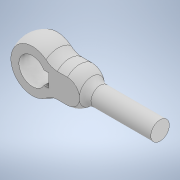
# Autodesk Inventor part: 1_3
Saved by Autodesk Inventor 2020.1 (Build 241239000, 239)
## iProperties
Created: 2022-02-23
Part Number: 1_3
Material: Типовые
Document SubType Name: Modeling
Designer: User
Density: 1 g/cm^3
Appearance: По умолчанию
Author: User
Autodesk Inventor part; units mm, degrees
ref_plane "YZ Plane" through (0, 0, 0) normal (1, 0, 0) x (0, 1, 0)
ref_plane "XZ Plane" through (0, 0, 0) normal (0, 1, 0) x (-1, 0, 0)
ref_plane "XY Plane" through (0, 0, 0) normal (0, 0, 1) x (1, 0, 0)
sketch "Эскиз1" plane through (0, 0, 0) normal (0, 0, 1) x (1, 0, 0)
  circle A0 centre (0, 0) radius 60
  circle A1 centre (0, 0) radius 32.5
  line L0 (28.2887, 16) -> (28.2887, -16)
  line L1 (28.2887, 16) -> (39.5, 16)
  line L2 (39.5, 16) -> (39.5, -16)
  line L3 (39.5, -16) -> (28.2887, -16)
  line L4 (-60, 0) -> (279.451, 0)
  line L5 (42.8486, 42) -> (42.8486, -42)
  line L6 (42.8486, 42) -> (85, 42)
  line L7 (85, 42) -> (85, -42)
  line L8 (85, -42) -> (42.8486, -42)
  line L9 (42.8486, -42) -> (42.8486, 42)
  circle A2 centre (60.2993, 92) radius 50
  line L10 (0, 0) -> (60.2993, 92)
  circle A3 centre (85, 0) radius 42
  line L11 (85, 22.5) -> (278.9533, 22.5)
  line L12 (278.9533, 22.5) -> (278.9533, -22.5)
  line L13 (278.9533, -22.5) -> (85, -22.5)
  line L14 (85, -22.5) -> (85, 22.5)
  circle A4 centre (134.2722, 52.5) radius 30
  line L15 (85, 0) -> (134.2722, 52.5)
  point P0 (-32.5, 0)
  point P1 (278.9533, 0)
  point P2 (278.9533, 0)
  point P3 (134.2722, 22.5)
  point P4 (113.7421, 30.625)
  point P5 (60.2993, 42)
  point P6 (32.8905, 50.1818)
  dimension "d17" = 84
  dimension "d0" = 120
  dimension "d1" = 65
  dimension "d2" = 32
  dimension "d3" = 72
  dimension "d4" = 84
  dimension "d7" = 100
  dimension "d8" = 92
  dimension "d10" = 110
  dimension "d11" = 85
  dimension "d12" = 0
  dimension "d13" = 45
  dimension "d14" = 60
  dimension "d15" = 52.5
  dimension "d16" = 72
  dimension "d18" = 0
  constraints: 32 end point, 6 point on circle, 5 horizontal, 5 parallel, 4 centre point, 4 perpendicular, 2 coincident, 2 midpoint, 2 point on line, 1 vertical, 3 other
  measures "d0" diameter of A0
  measures "d1" diameter of A1
  measures "d2" distance of L0.start L0.end
  measures "d3" horizontal distance of point (-32.5, 0) L1.end
  measures "d4" distance of L5.start L5.end
  measures "d7" diameter of A2
  measures "d8" distance from line of L4 L10.end
  measures "d10" distance of L10.start L10.end
  measures "d11" horizontal distance of L7.end point (0, 0)
  measures "d12" distance from line of L4 point (278.953, 0)
  measures "d13" distance of L11.end L12.end
  measures "d14" diameter of A4
  measures "d15" distance from line of L4 L15.end
  measures "d16" distance of L15.start L15.end
  measures "d18" distance of point (85, 0) L15.start
revolve "Вращение1" add sketch "Эскиз1" angle 360 about axis through (-60, 0, 0) along (1, 0, 0) picked at (45.8038, 26.0598) picked at (54.3043, 5.6582) picked at (76.4143, 10.6672) picked at (29.0608, 8.9784) contours A0 L10 A1 L4 | A2 L6 A0 | A0 L5 L4 L2 L1 A1 L10 | A1 L10 L4 | L5 A0 A3 L4 | L6 A3 A0 | A1 L0 L4 L10 | L4 A3 A0 | A0 A3 L7 L4 | L4 A1 L1 L2 | A3 L15 L11 L7 | A1 L4 L0 | L15 L11 A3 L4 | L7 L11 L15 | A3 L11 L12 L4 | A4 L11 A3 | A3 L11 L15
sketch "Эскиз2" plane through (0, 0, 0) normal (0, 1, 0) x (-1, 0, 0)
  line L0 (105.3756, -30) -> (-295.1428, -30)
  line L1 (-295.1428, -30) -> (-295.1428, 30)
  line L2 (-295.1428, 30) -> (105.3756, 30)
  line L3 (105.3756, 30) -> (105.3756, -30)
  point P0 (0, 0)
  point P1 (105.3756, 0)
  point P2 (0, 0)
  dimension "d20" = 0
  dimension "d21" = 60
  constraints: 8 end point, 2 parallel, 1 coincident, 1 horizontal, 1 midpoint, 1 perpendicular
  measures "d20" vertical distance of point (105.376, 0) point (0, 0)
  measures "d21" distance of L2.end L0.start
extrude "Выдавливание1" cut sketch "Эскиз2" along normal mid plane 200 keep common part
sketch "Эскиз3" plane through (60.2993, -29.3939, 30) normal (0, 0, 1) x (1, 0, 0)
  circle A0 centre (-60.2993, 29.3939) radius 32.5
  line L0 (-32.0106, 13.3939) -> (-32.0106, 45.3939)
  line L1 (-32.0106, 45.3939) -> (-20.7993, 45.3939)
  line L2 (-20.7993, 45.3939) -> (-20.7993, 13.3939)
  line L3 (-20.7993, 13.3939) -> (-32.0106, 13.3939)
  line L4 (-32.0106, 13.3939) -> (-32.0106, 45.3939)
  point P0 (-92.7993, 29.3939)
  point P1 (-32.0106, 13.3939)
  dimension "d24" = 65
  dimension "d25" = 32
  dimension "d26" = 72
  constraints: 10 end point, 3 point on circle, 2 parallel, 1 centre point, 1 coincident, 1 horizontal, 1 perpendicular, 1 vertical
  measures "d24" diameter of A0
  measures "d25" distance of L0.start L0.end
  measures "d26" horizontal distance of L2.end point (-92.799, 29.394)
extrude "Выдавливание2" cut sketch "Эскиз3" against normal blind 100
